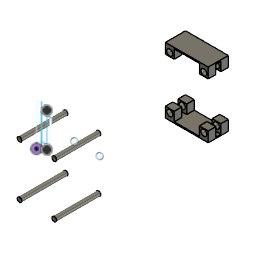
Camera Support (Autodesk Fusion 360 design; units mm, degrees)
part number: 2026-05-31-14-32-38-069
Autodesk Fusion 360 part; units mm, degrees
note: some values were not read from the file. Set by a fixed rule: which sketch regions a step uses.
sketch "Sketch10" plane through (0, 0, 0) normal (0, 0, 1) x (1, 0, 0)
  line L0 (0, 0) -> (5.6, 0)
  line L1 (5.6, 0) -> (5.6, 17)
  line L2 (5.6, 17) -> (0, 17)
  line L3 (0, 17) -> (0, 0)
  circle A0 centre (4.1311, 15.2456) radius 1.2
  line L4 (4.1311, 15.2456) -> (4.1311, 1.7456)
  circle A1 centre (4.1311, 1.7456) radius 1.2
  line L5 (5.6, 13.5027) -> (2, 13.5027)
  line L6 (2, 13.5027) -> (2, 3.5)
  line L7 (2, 3.5) -> (5.6, 3.5)
  line L8 (5.6, 3.5) -> (5.6, 13.5027)
  line L9 (2, 17) -> (2, 0)
  dimension "d71" = 5.6
  dimension "d72" = 17
  dimension "d73" = 2.4
  dimension "d74" = 13.5
  dimension "d75" = 2.4
  constraint horizontal L0
  constraint vertical L1
  constraint horizontal L2
  constraint vertical L3
  constraint coincident L0.start L3.end
  constraint coincident A0.centre L4.start
  constraint parallel L1 L4
  constraint coincident L4.end A1.centre
  constraint horizontal L5
  constraint vertical L6
  constraint horizontal L7
  constraint vertical L8
  constraint coincident L1 L5.start
  constraint coincident L2 L9.start
  constraint coincident L0 L9.end
  constraint perpendicular L0 L9
  measures "d71" distance of L0.start L0.end
  measures "d72" distance of L0.start L2.end
  measures "d73" diameter of A0
  measures "d74" distance of A0.centre L4.end
  measures "d75" diameter of A1
extrude "Extrude21" add sketch "Sketch10" against normal blind 4 contours L0 L2 L3 L6 L9 | L0 L1 L7 L9 | L1 L2 L5 L9 makes body 1
extrude "Extrude22" add sketch "Sketch10" along normal blind 4 contours L0 L2 L3 L6 L9 | L0 L1 L7 L9 | L1 L2 L5 L9 bodies 1
extrude "Extrude23" cut sketch "Sketch10" against normal blind 1 contours L0 L1 L7 L9 | L1 L2 L5 L9 bodies 1
extrude "Extrude24" cut sketch "Sketch10" along normal blind 1 contours L0 L1 L7 L9 | L1 L2 L5 L9 bodies 1
sketch "Sketch11" plane through (0, 0, 0) normal (0, 0, 1) x (1, 0, 0)
  circle A0 centre (15, 10) radius 0.95
  circle A1 centre (25, 10) radius 0.95
  dimension "d88" = 1.9
  dimension "d89" = 1.9
  measures "d88" diameter of A0
  measures "d89" diameter of A1
move_body "Move3" bodies 1 to x (1, 0, 0) y (0, 1, 0) z (0, 0, 1) at (0, 0, 4)
extrude "Extrude25" add sketch "Sketch11" along normal blind 10 separate body makes body 2 at (24.9763, 10.9497, 6.6667) makes body 3 at (15.9488, 9.9526, 6.6667)
extrude "Extrude26" add 1 faces at (14.7475, 9.7187, 10) along direction (0, 0, 1) blind 15 on bodies 3 bodies 3
extrude "Extrude27" add 1 faces at (24.6974, 10.1815, 10) along direction (0, 0, 1) blind 15 on bodies 2 bodies 2
copy_body "CopyPasteBodies1" bodies 1 2 3 makes body 4 makes body 5 makes body 6
move_body "Move4" bodies 4 5 6 to x (1, 0, 0) y (0, 1, 0) z (0, 0, 1) at (50, 0, 0)
move_body "Move5" bodies 6 4 5 to x (-1, 0, 0) y (0, -1, 0) z (0, 0, 1) at (128.1, 18.1, 0)
move_body "Move6" bodies 1 to x (0, 1, 0) y (-1, 0, 0) z (0, 0, 1) at (27, -9, -56)
move_body "Move7" bodies 1 to x (1, 0, 0) y (0, 1, 0) z (0, 0, 1) at (0, 0, -1.8)
move_body "Move8" bodies 1 to x (1, 0, 0) y (0, 1, 0) z (0, 0, 1) at (0, -5, 0)
extrude "Extrude28" cut 1 faces at (15.6667, -14, -55.1333) along direction (0, 1, 0) blind 1 on bodies 1 bodies 1
extrude "Extrude29" cut 1 faces at (78.1, 6.7667, 2.6667) along direction (-1, 0, 0) blind 1 on bodies 4 bodies 4
extrude "Extrude30" cut 1 faces at (77.1, 6.7667, 2.6667) along direction (-1, 0, 0) blind 0.5 on bodies 4 bodies 4
extrude "Extrude31" cut 1 faces at (15.6667, -13, -55.1333) along direction (0, 1, 0) blind 0.5 on bodies 1 bodies 1
move_body "Move9" bodies 1 to x (1, 0, 0) y (0, 1, 0) z (0, 0, 1) at (0, -1, 0)
move_body "Move10" bodies 4 to x (0, 1, 0) y (-1, 0, 0) z (0, 0, 1) at (20.6, -71.4, -59)
move_body "Move11" bodies 4 to x (1, 0, 0) y (0, 1, 0) z (0, 0, 1) at (0, 9, 1)
move_body "Move12" bodies 1 to x (1, 0, 0) y (0, 1, 0) z (0, 0, 1) at (0, -1, 57.8)
move_body "Move13" bodies 1 to x (1, 0, 0) y (0, 1, 0) z (0, 0, 1) at (0, 0, -58)
move_body "Move14" bodies 1 to x (1, 0, 0) y (0, 1, 0) z (0, 0, 1) at (-8, 24, 0)
move_body "Move15" bodies 4 to x (1, 0, 0) y (0, 1, 0) z (0, 0, 1) at (-0.5, 0, 0)
move_body "Move16" bodies 1 to x (1, 0, 0) y (0, 1, 0) z (0, 0, 1) at (0, 4.7, 0)
move_body "Move17" bodies 1 to x (1, 0, 0) y (0, 1, 0) z (0, 0, 1) at (0, -0.5, 0)
move_body "Move18" bodies 1 to x (1, 0, 0) y (0, 1, 0) z (0, 0, 1) at (0, -25, 0)
move_body "Move19" bodies 1 to x (1, 0, 0) y (0, 1, 0) z (0, 0, 1) at (0, -0.5, 0)
move_body "Move20" bodies 4 1 2 3 to x (1, 0, 0) y (0, 1, 0) z (0, 0, 1) at (0, -1, 0)
move_body "Move21" bodies 1 3 2 4 to x (1, 0, 0) y (0, 1, 0) z (0, 0, 1) at (0, -0.5, 0)
move_body "Move22" bodies 1 2 4 3 to x (1, 0, 0) y (0, 1, 0) z (0, 0, 1) at (0, 0.5, 0)
move_body "Move23" bodies 1 2 4 3 to x (1, 0, 0) y (0, 1, 0) z (0, 0, 1) at (0, 5.8913, 0)
move_body "Move24" bodies 1 2 4 3 to x (1, 0, 0) y (0, 1, 0) z (0, 0, 1) at (0, 6.9087, 0)
move_body "Move25" bodies 1 2 4 3 to x (1, 0, 0) y (0, 1, 0) z (0, 0, 1) at (0, -13, 0)
move_body "Move26" bodies 3 2 to x (1, 0, 0) y (0, 1, 0) z (0, 0, 1) at (-10.2512, 0, -53)
move_body "Move27" bodies 3 2 to x (1, 0, 0) y (0, 1, 0) z (0, 0, 1) at (-1, 1.6, 0)
move_body "Move28" bodies 2 to x (1, 0, 0) y (0, 1, 0) z (0, 0, 1) at (3.5, 0, 0)
move_body "Move29" bodies 5 6 to x (1, 0, 0) y (0, 1, 0) z (0, 0, 1) at (-48.3, -18.45, -50)
move_body "Move30" bodies 5 6 to x (1, 0, 0) y (0, 1, 0) z (0, 0, 1) at (-1.1012, 0, 0)
move_body "Move31" bodies 5 to x (1, 0, 0) y (0, 1, 0) z (0, 0, 1) at (0.0513, 0, 22)
move_body "Move32" bodies 5 to x (1, 0, 0) y (0, 1, 0) z (0, 0, 1) at (0, 0, -28)
move_body "Move33" bodies 2 to x (1, 0, 0) y (0, 1, 0) z (0, 0, 1) at (0, -0.05, 0)
move_body "Move34" bodies 3 to x (1, 0, 0) y (0, 1, 0) z (0, 0, 1) at (0, -0.05, 0)
move_body "Move35" bodies 6 to x (1, 0, 0) y (0, 1, 0) z (0, 0, 1) at (3.55, 0, -8)
move_body "Move36" bodies 2 to x (1, 0, 0) y (0, 1, 0) z (0, 0, 1) at (0, 0, 19)
move_body "Move37" bodies 2 to x (1, 0, 0) y (0, 1, 0) z (0, 0, 1) at (0, 0, 20.5)
move_body "Move38" bodies 2 to x (1, 0, 0) y (0, 1, 0) z (0, 0, 1) at (0, 0, -1)
move_body "Move39" bodies 2 to x (1, 0, 0) y (0, 1, 0) z (0, 0, 1) at (0, 0, -1)
move_body "Move40" bodies 2 to x (1, 0, 0) y (0, 1, 0) z (0, 0, 1) at (0, 0, 0.5)
move_body "Move41" bodies 2 to x (1, 0, 0) y (0, 1, 0) z (0, 0, 1) at (0, 0, 0.25)
extrude "Extrude32" cut 1 faces at (16.9462, 10.5315, -14.75) along direction (0, 0, 1) blind 4 on bodies 2 bodies 2
extrude "Extrude33" cut 1 faces at (16.9462, 10.5315, -10.75) along direction (0, 0, 1) blind 0.5 on bodies 2 bodies 2
move_body "Move42" bodies 3 to x (1, 0, 0) y (0, 1, 0) z (0, 0, 1) at (0, 0, 39)
move_body "Move43" bodies 3 to x (1, 0, 0) y (0, 1, 0) z (0, 0, 1) at (0, 0, -1)
move_body "Move44" bodies 3 to x (1, 0, 0) y (0, 1, 0) z (0, 0, 1) at (0, 0, 0.5)
extrude "Extrude34" cut 1 faces at (3.5486, 10.8602, -14.5) along direction (0, 0, 1) blind 3 on bodies 3 bodies 3
move_body "Move45" bodies 3 to x (1, 0, 0) y (0, 1, 0) z (0, 0, 1) at (0, 0, 0.5)
move_body "Move46" bodies 3 to x (1, 0, 0) y (0, 1, 0) z (0, 0, 1) at (0, 0, -1)
extrude "Extrude35" cut 1 faces at (3.5486, 10.8602, -12) along direction (0, 0, 1) blind 1 on bodies 3 bodies 3
move_body "Move47" bodies 3 to x (1, 0, 0) y (0, 1, 0) z (0, 0, 1) at (0, 0, -1)
move_body "Move48" bodies 3 to x (1, 0, 0) y (0, 1, 0) z (0, 0, 1) at (0, 0, 1)
move_body "Move49" bodies 3 to x (1, 0, 0) y (0, 1, 0) z (0, 0, 1) at (0, 0, 0.5)
extrude "Extrude36" cut 1 faces at (3.5486, 10.8602, -10.5) along direction (0, 0, 1) blind 2.7 on bodies 3 bodies 3
extrude "Extrude37" cut 1 faces at (16.9462, 10.5315, -10.25) along direction (0, 0, 1) blind 2.9 on bodies 2 bodies 2
move_body "Move50" bodies 6 to x (1, 0, 0) y (0, 1, 0) z (0, 0, 1) at (0, 0, 12)
move_body "Move51" bodies 5 to x (1, 0, 0) y (0, 1, 0) z (0, 0, 1) at (0, 0, 10)
extrude "Extrude38" cut 1 faces at (17.3192, -10.6587, -21) along direction (0, 0, -1) blind 7.4 on bodies 6 bodies 6
extrude "Extrude39" cut 1 faces at (3.5179, -10.6598, -21) along direction (0, 0, -1) blind 6.7 on bodies 5 bodies 5
move_body "Move52" bodies 6 to x (1, 0, 0) y (0, 1, 0) z (0, 0, 1) at (0, 0, 38.65)
move_body "Move53" bodies 5 to x (1, 0, 0) y (0, 1, 0) z (0, 0, 1) at (0, 0, 38.2)
move_body "Move54" bodies 1 to x (1, 0, 0) y (0, 1, 0) z (0, 0, 1) at (0, 0, 1)
move_body "Move55" bodies 4 to x (1, 0, 0) y (0, 1, 0) z (0, 0, 1) at (0, 0, 1)
